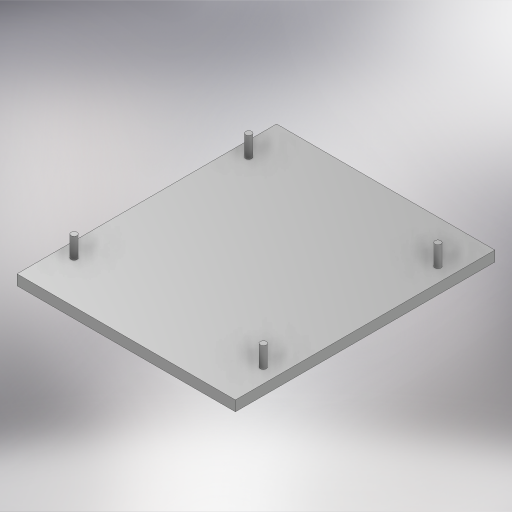
# Autodesk Inventor part: Tapa 0
Saved by Autodesk Inventor 2024 (Build 280153000, 153)
## iProperties
Created: 2023-11-10
Part Number: Tapa 0
Material: Genérico
Document SubType Name: Modeling
Designer: juesr
Density: 1 g/cm^3
Appearance: Valor por defecto
Author: juesr
Autodesk Inventor part; units mm, degrees
ref_plane "YZ Plane" through (0, 0, 0) normal (1, 0, 0) x (0, 1, 0)
ref_plane "XZ Plane" through (0, 0, 0) normal (0, 1, 0) x (-1, 0, 0)
ref_plane "XY Plane" through (0, 0, 0) normal (0, 0, 1) x (1, 0, 0)
sketch "Boceto1" plane through (0, 0, 0) normal (0, 1, 0) x (-1, 0, 0)
  line L0 (53, 63) -> (-53, 63)
  line L1 (-53, 63) -> (-53, -63)
  line L2 (-53, -63) -> (53, -63)
  line L3 (53, -63) -> (53, 63)
  point P0 (0, 0)
  point P1 (0, 63)
  dimension "d1" = 106
  dimension "d2" = 126
  dimension "d3" = 53
  dimension "d4" = 63
  constraints: 8 end point, 2 parallel, 1 horizontal, 1 midpoint, 1 perpendicular
  measures "d1" distance between parallel lines of L1 L3
  measures "d2" distance between parallel lines of L2 L0
  measures "d3" distance from line of L3 point (0, 0)
  measures "d4" distance of point (0, 63) point (0, 0)
extrude "Extrusión1" add sketch "Boceto1" along normal blind 5
sketch "Boceto2" plane through (0, 5, 0) normal (0, 1, 0) x (1, 0, 0)
  circle A0 centre (-45.929, -42.384) radius 1.5
  line L0 (-53, -63) -> (53, -63) projected
  line L1 (-53, 63) -> (-53, -63) projected
  line L2 (-81, 0) -> (77, 0)
  line L3 (0, -130) -> (0, 128)
  circle A1 centre (-45.929, 42.384) radius 1.5
  line L4 (-53, -63) -> (-53, 63)
  circle A2 centre (45.929, -42.384) radius 1.5
  circle A3 centre (45.929, 42.384) radius 1.5
  point P0 (0, 0)
  dimension "d7" = 3
  dimension "d8" = 20.616
  dimension "d9" = 7.071
  constraints: 6 end point, 5 symmetric about line, 4 centre point, 1 horizontal, 1 vertical, 3 other
  measures "d7" diameter of A0
  measures "d8" distance from line of L0 A0.centre
  measures "d9" distance from line of L1 A0.centre
extrude "Extrusión2" add sketch "Boceto2" along normal blind 10 contours A0 | A1 | A2 | A3
sketch "Boceto3" plane through (0, 0, 0) normal (0, -1, 0) x (1, 0, 0)
  line L0 (-35, 52.5) -> (35, 52.5)
  line L1 (35, 52.5) -> (35, -52.5)
  line L2 (35, -52.5) -> (-35, -52.5)
  line L3 (-35, -52.5) -> (-35, 52.5)
  line L4 (53, -63) -> (-53, -63) projected
  line L5 (-53, 63) -> (53, 63) projected
  line L6 (53, 63) -> (53, -63) projected
  line L7 (-53, -63) -> (-53, 63) projected
  line L8 (35, 17.5) -> (-35, 17.5)
  line L9 (35, -17.5) -> (-35, -17.5)
  line L10 (0, 52.5) -> (0, -52.5)
  point P0 (0, 0)
  point P1 (0, 17.5)
  point P2 (0, -17.5)
  dimension "d12" = 52.5
  dimension "d13" = 126
  dimension "d14" = 106
  dimension "d15" = 52.5
  dimension "d16" = 35
  dimension "d17" = 35
  dimension "d18" = 35
  dimension "d19" = 35
  dimension "d20" = 35
  constraints: 14 end point, 4 point on line, 3 perpendicular, 2 midpoint, 2 parallel, 1 horizontal
  measures "d12" distance of L10.start point (0, 0)
  measures "d13" distance between parallel lines of L4 L5
  measures "d14" distance between parallel lines of L6 L7
  measures "d15" distance from line of L2 point (0, 0)
  measures "d16" distance from line of L1 point (0, 0)
  measures "d17" distance from line of L3 point (0, 0)
  measures "d18" distance between parallel lines of L0 L8
  measures "d19" distance between parallel lines of L2 L9
  measures "d20" distance between parallel lines of L9 L8
extrude "Extrusión3" cut sketch "Boceto3" against normal blind 2 contours L0 L1 L8 L10 | L8 L10 L9 L3
